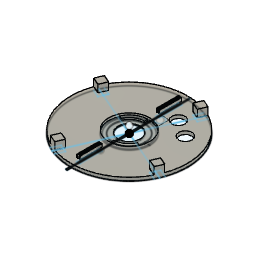
Capuchon TrapMonster v2 (Autodesk Fusion 360 design; units mm, degrees)
Autodesk Fusion 360 part; units mm, degrees
sketch "Sketch1" plane through (0, 0, 0) normal (0, 1, 0) x (1, 0, 0)
  circle A0 centre (0, 0) radius 13.5
  circle A1 centre (0, 0) radius 19.35
  circle A2 centre (0, 0) radius 19.5
  circle A3 centre (0, 0) radius 23.3
  circle A4 centre (0, 0) radius 71
  line L0 (0, 0) -> (0, 71)
  line L1 (0, 0) -> (0, -71)
  line L2 (0, 0) -> (0.77, 0)
  line L3 (0.77, 0) -> (0.77, -76)
  line L4 (0.77, -76) -> (0, -76)
  line L5 (0, -76) -> (0, 0)
  line L6 (0, 0) -> (-0.77, 0)
  line L7 (-0.77, 0) -> (-0.77, -76)
  line L8 (-0.77, -76) -> (0, -76)
  line L9 (0, -76) -> (0, 0)
  line L10 (-0.77, 0) -> (0, 0)
  line L11 (0, 0) -> (0, 73)
  line L12 (0, 73) -> (-0.77, 73)
  line L13 (-0.77, 73) -> (-0.77, 0)
  line L14 (0, 73) -> (0.77, 73)
  line L15 (0.77, 73) -> (0.77, 0)
  line L16 (0.77, 0) -> (0, 0)
  line L17 (0, 0) -> (0, 73)
  line L18 (0, 0) -> (0, 35)
  line L19 (0, 0) -> (0, -35)
  line L20 (-0.77, 35) -> (-2, 35)
  line L21 (-2, 35) -> (-2, 62)
  line L22 (-2, 62) -> (-0.77, 62)
  line L23 (-0.77, 62) -> (-0.77, 35)
  line L24 (0.77, 35) -> (2, 35)
  line L25 (2, 35) -> (2, 62)
  line L26 (2, 62) -> (0.77, 62)
  line L27 (0.77, 62) -> (0.77, 35)
  line L28 (0.77, -35.0032) -> (2, -35.0032)
  line L29 (2, -35.0032) -> (2, -62)
  line L30 (2, -62) -> (0.77, -62)
  line L31 (0.77, -62) -> (0.77, -35.0032)
  line L32 (-0.77, -34.7868) -> (-2, -34.7868)
  line L33 (-2, -34.7868) -> (-2, -62)
  line L34 (-2, -62) -> (-0.77, -62)
  line L35 (-0.77, -62) -> (-0.77, -34.7868)
  line L36 (0, 0) -> (65.1081, -28.3184)
  line L37 (0, 0) -> (-28.3184, -65.1081)
  line L38 (-28.3184, -65.1081) -> (28.3184, 65.1081)
  line L39 (28.3184, 65.1081) -> (24.3299, 55.938)
  line L40 (0, 0) -> (-65.1081, 28.3184)
  line L41 (-65.1081, 28.3184) -> (-55.938, 24.3299)
  line L42 (65.1081, -28.3184) -> (55.938, -24.3299)
  line L43 (-28.3184, -65.1081) -> (-24.3299, -55.938)
  line L44 (-55.938, 24.3299) -> (-53.9437, 28.9149)
  line L45 (24.3299, 55.938) -> (28.9149, 53.9437)
  line L46 (55.938, -24.3299) -> (57.9322, -19.7448)
  line L47 (-24.3299, -55.938) -> (-19.7448, -57.9322)
  line L48 (-53.9437, 28.9149) -> (-62.9522, 32.8331)
  line L49 (-53.9437, 28.9149) -> (-57.9322, 19.7448)
  line L50 (-57.9322, 19.7448) -> (-66.9407, 23.663)
  line L51 (-24.3299, -55.938) -> (-28.9149, -53.9437)
  line L52 (-28.9149, -53.9437) -> (-32.8331, -62.9522)
  line L53 (-19.7448, -57.9322) -> (-23.663, -66.9407)
  line L54 (57.9322, -19.7448) -> (66.9407, -23.663)
  line L55 (55.938, -24.3299) -> (53.9437, -28.9149)
  line L56 (53.9437, -28.9149) -> (62.9522, -32.8331)
  line L57 (28.9149, 53.9437) -> (32.8331, 62.9522)
  line L58 (24.3299, 55.938) -> (19.7448, 57.9322)
  line L59 (19.7448, 57.9322) -> (23.663, 66.9407)
  circle A5 centre (0, 0) radius 25
  dimension "d1" = 27
  dimension "d2" = 38.7
  dimension "d3" = 39
  dimension "d4" = 46.6
  dimension "d5" = 142
  dimension "d6" = 0.77
  dimension "d7" = 0.77
  dimension "d8" = 35
  dimension "d9" = 35
  dimension "d10" = 10
  dimension "d11" = 10
  dimension "d12" = 10
  dimension "d13" = 10
  dimension "d14" = 5
  dimension "d15" = 5
  dimension "d16" = 5
  dimension "d17" = 5
  dimension "d18" = 10
  dimension "d19" = 5
  dimension "d20" = 5
  dimension "d21" = 5
  dimension "d22" = 50
  constraint coincident A0.centre A1.centre
  constraint concentric A2 A3
  constraint coincident A4 L0.end
  constraint vertical L0
  constraint coincident A4 L1.end
  constraint parallel L0 L1
  constraint horizontal L2
  constraint vertical L3
  constraint horizontal L4
  constraint vertical L5
  constraint horizontal L6
  constraint vertical L7
  constraint horizontal L8
  constraint vertical L9
  constraint horizontal L10
  constraint vertical L11
  constraint horizontal L12
  constraint vertical L13
  constraint horizontal L14
  constraint vertical L15
  constraint horizontal L16
  constraint vertical L17
  constraint coincident L17 L18.end
  constraint coincident L0 L18.end
  constraint perpendicular L6 L19
  constraint horizontal L20
  constraint vertical L21
  constraint horizontal L22
  constraint vertical L23
  constraint coincident L13 L20.start
  constraint horizontal L24
  constraint vertical L25
  constraint horizontal L26
  constraint vertical L27
  constraint coincident L15 L24.start
  constraint horizontal L28
  constraint vertical L29
  constraint horizontal L30
  constraint vertical L31
  constraint coincident L3 L28.start
  constraint horizontal L32
  constraint vertical L33
  constraint horizontal L34
  constraint vertical L35
  constraint coincident L7 L32.start
  constraint coincident A4 L36.end
  constraint coincident A4 L37.end
  constraint perpendicular L36 L37
  constraint coincident A4 L38.end
  constraint parallel L37 L38
  constraint parallel L38 L39
  constraint coincident A4 L40.end
  constraint perpendicular L37 L40
  constraint parallel L40 L41
  constraint parallel L36 L42
  constraint parallel L37 L43
  constraint perpendicular L40 L44
  constraint perpendicular L39 L45
  constraint perpendicular L42 L46
  constraint perpendicular L43 L47
  constraint coincident A4 L48.end
  constraint perpendicular L44 L48
  constraint perpendicular L48 L49
  constraint coincident A4 L50.end
  constraint perpendicular L49 L50
  constraint perpendicular L43 L51
  constraint coincident A4 L52.end
  constraint perpendicular L51 L52
  constraint coincident A4 L53.end
  constraint perpendicular L47 L53
  constraint coincident A4 L54.end
  constraint perpendicular L46 L54
  constraint perpendicular L36 L55
  constraint coincident A4 L56.end
  constraint perpendicular L55 L56
  constraint coincident A4 L57.end
  constraint perpendicular L45 L57
  constraint perpendicular L38 L58
  constraint coincident A4 L59.end
  constraint perpendicular L58 L59
  measures "d1" diameter of A0
  measures "d2" diameter of A1
  measures "d3" diameter of A2
  measures "d4" diameter of A3
  measures "d5" diameter of A4
  measures "d6" distance of A0.centre L2.end
  measures "d7" distance of A0.centre L6.end
  measures "d8" distance of A0.centre L18.end
  measures "d9" distance of A0.centre L19.end
  measures "d10" distance of L38.end L39.end
  measures "d11" distance of L40.end L41.end
  measures "d12" distance of L36.end L42.end
  measures "d13" distance of L37.end L43.end
  measures "d14" distance of L41.end L44.end
  measures "d15" distance of L39.end L45.end
  measures "d16" distance of L42.end L46.end
  measures "d17" distance of L43.end L47.end
  measures "d18" distance of L44.end L49.end
  measures "d19" distance of L43.end L51.end
  measures "d20" distance of L42.end L55.end
  measures "d21" distance of L39.end L58.end
  measures "d22" diameter of A5
extrude "Extrude1" add sketch "Sketch1" along normal blind 3 contours A4 L15 L24 L25 L26 L38 L58 L59 A5 | A4 L36 L38 L45 L46 L54 L57 A5 | A4 L3 L28 L29 L30 L36 L55 L56 A5 | A4 L0 L11 L15 L17 L18 L27 A5 | A4 L38 L39 L58 L59 | A4 L38 L39 L45 L57 | A4 L1 L3 L5 L9 L19 L31 A5 | A4 L36 L42 L46 L54 | A4 L36 L42 L55 L56 | A4 L0 L11 L13 L17 L18 L23 A5 | L15 L24 L25 L26 L27 | A4 L1 L5 L7 L9 L19 L35 A5 | L3 L28 L29 L30 L31 | A4 L13 L20 L21 L22 L40 L44 L48 L49 A5 | A4 L7 L32 L33 L34 L37 L38 L47 L53 A5 | A4 L37 L38 L40 L49 L50 L51 L52 A5 | L13 L20 L21 L22 L23 | L7 L32 L33 L34 L35 | A4 L40 L41 L49 L50 | A4 L40 L41 L44 L48 L49 | A4 L37 L38 L43 L47 L53 | A4 L37 L38 L43 L51 L52
extrude "Extrude2" add sketch "Sketch1" along normal blind 13 contours A4 L38 L39 L58 L59 | A4 L38 L39 L45 L57 | A4 L36 L42 L46 L54 | A4 L36 L42 L55 L56 | A4 L40 L41 L49 L50 | A4 L40 L41 L44 L48 L49 | A4 L37 L38 L43 L47 L53 | A4 L37 L38 L43 L51 L52
extrude "Extrude3" add sketch "Sketch1" along normal blind 8 contours L15 L24 L25 L26 L27 | L3 L28 L29 L30 L31 | L13 L20 L21 L22 L23 | L7 L32 L33 L34 L35
extrude "Extrude4" add 1 faces at (37.708, 3, 34.8341) along direction (0, 1, 0) blind 1
sketch "Sketch2" plane through (0, 4, 0) normal (0, 1, 0) x (-1, 0, 0)
  line L0 (-0.77, -62) -> (-2, -62)
  line L1 (-2, -62) -> (-2, -35)
  line L2 (-2, -35) -> (-0.77, -35)
  line L3 (-0.77, -35) -> (-0.77, -62)
  line L4 (0.77, 62) -> (2, 62)
  line L5 (2, 62) -> (2, 34.7868)
  line L6 (2, 34.7868) -> (0.77, 34.7868)
  line L7 (0.77, 34.7868) -> (0.77, 62)
  line L8 (0.77, -62) -> (0.77, -35)
  line L9 (0.77, -35) -> (2, -35)
  line L10 (2, -35) -> (2, -62)
  line L11 (2, -62) -> (0.77, -62)
  line L12 (-0.77, 62) -> (-0.77, 35.0032)
  line L13 (-0.77, 35.0032) -> (-2, 35.0032)
  line L14 (-2, 35.0032) -> (-2, 62)
  line L15 (-2, 62) -> (-0.77, 62)
  circle A0 centre (0, 0) radius 25
  line L16 (-62.9522, 32.8331) -> (-53.9437, 28.9149)
  line L17 (-53.9437, 28.9149) -> (-57.9322, 19.7448)
  line L18 (-57.9322, 19.7448) -> (-66.9407, 23.663)
  arc A1 (-66.9407, 23.663) -> (-32.8331, -62.9522) centre (0, 0) ccw
  line L19 (-32.8331, -62.9522) -> (-28.9149, -53.9437)
  line L20 (-28.9149, -53.9437) -> (-19.7448, -57.9322)
  line L21 (-19.7448, -57.9322) -> (-23.663, -66.9407)
  arc A2 (-23.663, -66.9407) -> (62.9522, -32.8331) centre (0, 0) ccw
  line L22 (62.9522, -32.8331) -> (53.9437, -28.9149)
  line L23 (53.9437, -28.9149) -> (57.9322, -19.7448)
  line L24 (57.9322, -19.7448) -> (66.9407, -23.663)
  arc A3 (66.9407, -23.663) -> (32.8331, 62.9522) centre (0, 0) ccw
  line L25 (32.8331, 62.9522) -> (28.9149, 53.9437)
  line L26 (28.9149, 53.9437) -> (19.7448, 57.9322)
  line L27 (19.7448, 57.9322) -> (23.663, 66.9407)
  arc A4 (23.663, 66.9407) -> (-62.9522, 32.8331) centre (0, 0) ccw
  line L28 (0, 0) -> (-20, -40)
  circle A5 centre (-20, -40) radius 8
  line L29 (-20, -40) -> (-12.8446, -43.5777)
  line L30 (-20, -40) -> (-54.5328, -19.2256)
  line L31 (-26.8552, -35.8761) -> (-34.2244, -31.4428)
  line L32 (-34.2244, -31.4428) -> (-41.0796, -27.3189)
  circle A6 centre (-41.0796, -27.3189) radius 8
  dimension "d31" = 16
  dimension "d32" = 40.3
  dimension "d33" = 8.6
  dimension "d34" = 8
  dimension "d35" = 16
  constraint coincident A0.centre A1.centre
  constraint coincident L28.end A5.centre
  constraint coincident A5 L29.end
  constraint perpendicular L28 L29
  constraint coincident L30 L31.start
  constraint coincident A5 L31.start
  constraint parallel L30 L31
  constraint parallel L30 L32
  constraint coincident L32.end A6.centre
  measures "d31" diameter of A5
  measures "d32" distance of L28.end L30.end
  measures "d33" distance of L31.start L31.end
  measures "d34" distance of L31.end L32.end
  measures "d35" diameter of A6
extrude "Extrude5" cut sketch "Sketch2" against normal blind 36 contours L28 A5 L29 | L28 A5 L30 | A5 L29 L30 | L30 L32 A6 | L30 L32 A6
extrude "Extrude6" add sketch "Sketch1" along normal blind 1 contours A0 L3 L15 L36 L38 | A0 A1 L36 L38 | A0 L15 L38 | A0 A1 L15 L38 | A0 A1 L3 L36 | A0 L3 L36 | A0 L0 L11 L15 L17 L18 L38 | A0 A1 L0 L11 L15 L17 L18 | L2 L15 L16 L38 | A1 A2 L36 L38 | A1 A2 L15 L38 | A0 A1 L1 L3 L5 L9 L19 | A0 L1 L3 L5 L9 L19 L36 | L2 L3 L16 L36 | A1 A2 L3 L36 | A0 L0 L11 L13 L17 L18 L40 | A0 A1 L0 L11 L13 L17 L18 | A1 A2 L0 L11 L15 L17 L18 | L6 L7 L10 L37 L38 | A0 L1 L5 L7 L9 L19 L37 L38 | L6 L10 L13 L40 | A2 A3 L36 L38 | A2 A3 L15 L38 | A0 A1 L1 L5 L7 L9 L19 | A1 A2 L1 L3 L5 L9 L19 | A2 A3 L3 L36 | A0 L13 L40 | A0 A1 L13 L40 | A1 A2 L0 L11 L13 L17 L18 | A2 A3 L0 L11 L15 L17 L18 | A0 L7 L13 L37 L38 L40 | A0 L7 L37 L38 | A3 L36 L38 A5 | A3 L15 L38 A5 | A0 A1 L7 L37 L38 | A1 A2 L1 L5 L7 L9 L19 | A2 A3 L1 L3 L5 L9 L19 | A3 L3 L36 A5 | A0 A1 L37 L38 L40 | A1 A2 L13 L40 | A2 A3 L0 L11 L13 L17 L18 | A3 L0 L11 L15 L17 L18 A5 | A1 A2 L7 L37 L38 | A2 A3 L1 L5 L7 L9 L19 | A3 L1 L3 L5 L9 L19 A5 | A1 A2 L37 L38 L40 | A2 A3 L13 L40 | A3 L0 L11 L13 L17 L18 A5 | A2 A3 L7 L37 L38 | A3 L1 L5 L7 L9 L19 A5 | A2 A3 L37 L38 L40 | A3 L13 L40 A5 | A3 L7 L37 L38 A5 | A3 L37 L38 L40 A5
sketch "Sketch3" plane through (0, 0, 0) normal (0, 0, 1) x (1, 0, 0)
  line L0 (4.4303, 3.3085) -> (13.6469, 3.3085)
  line L1 (13.6469, 3.3085) -> (13.6469, 1.0043)
  line L2 (13.6469, 1.0043) -> (4.4303, 1.0043)
  line L3 (4.4303, 1.0043) -> (4.4303, 3.3085)
  constraint horizontal L0
  constraint vertical L1
  constraint horizontal L2
  constraint vertical L3
extrude "Extrude7" cut sketch "Sketch3" against normal blind 35
sketch "Sketch4" plane through (0, 1, 0) normal (0, 1, 0) x (-1, 0, 0)
  circle A0 centre (0, 0) radius 25
  circle A1 centre (-5.7905, -31.8479) radius 4.9823
sketch "Sketch5" plane through (0, 1, 0) normal (0, 1, 0) x (-1, 0, 0)
sketch "Sketch6" plane through (0, 0, 0) normal (0, 0, 1) x (1, 0, 0)
  circle A0 centre (0, 8.5) radius 1.5
  dimension "d42" = 3
  measures "d42" diameter of A0
extrude "Extrude8" cut sketch "Sketch1" along normal blind 28 contours A0 L3 L15 L36 L38 | A0 L15 L38 | A0 L3 L36 | A0 L0 L11 L15 L17 L18 L38 | L2 L15 L16 L38 | A0 L1 L3 L5 L9 L19 L36 | L2 L3 L16 L36 | A0 L0 L11 L13 L17 L18 L40 | L6 L7 L10 L37 L38 | A0 L1 L5 L7 L9 L19 L37 L38 | L6 L10 L13 L40 | A0 L13 L40 | A0 L7 L13 L37 L38 L40 | A0 L7 L37 L38
extrude "Extrude9" add sketch "Sketch1" along normal blind 3 contours A2 A3 L3 L36 | A2 A3 L13 L40
